Autodesk Inventor part; units mm, degrees
(part 2 of 2)
  spline S266 degree 2 poles (-40.3504, -60.3265) (-40.034, -60.3265) (-39.4952, -60.2771) (-39.3469, -60.198) knots 0 0 0 1 2 2 2
  spline S267 degree 2 poles (-39.3469, -60.198) (-39.1838, -60.1189) (-39.0256, -59.8173) (-39.0256, -59.5553) knots 0 0 0 1 2 2 2
  spline S268 degree 2 poles (-39.0256, -59.5553) (-39.0256, -59.3181) (-39.3173, -58.7743) (-39.5941, -58.4876) knots 0 0 0 1 2 2 2
  spline S269 degree 2 poles (-39.5941, -58.4876) (-39.6633, -58.4925) (-39.8561, -58.5024) (-39.9846, -58.5024) knots 0 0 0 1 2 2 2
  line L190 (-39.9846, -58.5024) -> (-43, -58.5024)
  line L191 (-43, -58.5024) -> (-43, -57.7313)
  line L192 (-43, -57.7313) -> (-40.3504, -57.7313)
  spline S270 degree 2 poles (-40.3504, -57.7313) (-40.034, -57.7313) (-39.4952, -57.6818) (-39.3469, -57.6028) knots 0 0 0 1 2 2 2
  spline S271 degree 2 poles (-39.3469, -57.6028) (-39.1838, -57.5237) (-39.0256, -57.2221) (-39.0256, -56.9601) knots 0 0 0 1 2 2 2
  spline S272 degree 2 poles (-39.0256, -56.9601) (-39.0256, -56.713) (-39.337, -56.1643) (-39.5793, -55.9072) knots 0 0 0 1 2 2 2
  line L193 (-39.5793, -55.9072) -> (-43, -55.9072)
  line L194 (-43, -55.9072) -> (-43, -55.1361)
  line L195 (-43, -55.1361) -> (-38.4225, -55.1361)
  line L196 (-38.4225, -55.1361) -> (-38.4225, -55.9072)
  line L197 (-38.4225, -55.9072) -> (-38.9267, -55.9072)
  spline S273 degree 2 poles (-38.9267, -55.9072) (-38.6252, -56.2088) (-38.294, -56.8019) (-38.294, -57.1579) knots 0 0 0 1 2 2 2
  spline S274 degree 2 poles (-38.294, -57.1579) (-38.294, -57.5632) (-38.6647, -58.191) (-39.0849, -58.3541) knots 0 0 0 1 2 2 2
  spline S275 degree 2 poles (-39.0849, -58.3541) (-38.6944, -58.7051) (-38.294, -59.3675) (-38.294, -59.7531) knots 0 0 0 1 2 2 2
  spline S276 degree 2 poles (-38.294, -59.7531) (-38.294, -60.0497) (-38.4769, -60.5341) (-38.6845, -60.7121) knots 0 0 0 1 2 2 2
  spline S277 degree 2 poles (-38.6845, -60.7121) (-38.8921, -60.895) (-39.515, -61.0976) (-39.9846, -61.0976) knots 0 0 0 1 2 2 2
  line L198 (-39.9846, -61.0976) -> (-43, -61.0976)
  line L199 (-43, -61.0976) -> (-43, -60.3265)
  spline S278 degree 2 poles (-53.1384, -40.6671) (-53.1384, -40.2123) (-52.8665, -39.4659) (-52.6144, -39.2039) knots 0 0 0 1 2 2 2
  spline S279 degree 2 poles (-52.6144, -39.2039) (-52.3673, -38.9468) (-51.695, -38.6799) (-51.3143, -38.6799) knots 0 0 0 1 2 2 2
  spline S280 degree 2 poles (-51.3143, -38.6799) (-50.82, -38.6799) (-49.9895, -39.2088) (-49.7424, -39.713) knots 0 0 0 1 2 2 2
  line L200 (-49.7424, -39.713) -> (-49.7177, -39.713)
  spline S281 degree 2 poles (-49.7177, -39.713) (-49.4557, -39.2632) (-48.8328, -38.8282) (-48.3682, -38.8282) knots 0 0 0 1 2 2 2
  spline S282 degree 2 poles (-48.3682, -38.8282) (-47.681, -38.8282) (-46.7616, -39.8663) (-46.7616, -40.6671) knots 0 0 0 1 2 2 2
  spline S283 degree 2 poles (-46.7616, -40.6671) (-46.7616, -41.4976) (-47.6316, -42.5011) (-48.3138, -42.5011) knots 0 0 0 1 2 2 2
  spline S284 degree 2 poles (-48.3138, -42.5011) (-48.7241, -42.5011) (-49.5249, -42.0216) (-49.7523, -41.5717) knots 0 0 0 1 2 2 2
  line L201 (-49.7523, -41.5717) -> (-49.777, -41.5717)
  spline S285 degree 2 poles (-49.777, -41.5717) (-50.0241, -42.1056) (-50.736, -42.6543) (-51.2995, -42.6543) knots 0 0 0 1 2 2 2
  spline S286 degree 2 poles (-51.2995, -42.6543) (-52.0806, -42.6543) (-53.1384, -41.5173) (-53.1384, -40.6671) knots 0 0 0 1 2 2 2
  spline S287 degree 2 poles (-51.3786, -41.8139) (-51.0029, -41.8139) (-50.558, -41.5173) (-50.3306, -41.0972) knots 0 0 0 1 2 2 2
  spline S288 degree 2 poles (-50.3306, -41.0972) (-50.2515, -40.9588) (-50.0686, -40.4941) (-49.95, -40.2024) knots 0 0 0 1 2 2 2
  spline S289 degree 2 poles (-49.95, -40.2024) (-50.1724, -39.8663) (-50.8348, -39.5054) (-51.255, -39.5054) knots 0 0 0 1 2 2 2
  spline S290 degree 2 poles (-51.255, -39.5054) (-51.8087, -39.5054) (-52.5304, -40.1728) (-52.5304, -40.677) knots 0 0 0 1 2 2 2
  spline S291 degree 2 poles (-52.5304, -40.677) (-52.5304, -41.1911) (-51.9125, -41.8139) (-51.3786, -41.8139) knots 0 0 0 1 2 2 2
  spline S292 degree 2 poles (-48.3237, -41.7002) (-47.9134, -41.7002) (-47.3647, -41.1515) (-47.3647, -40.6622) knots 0 0 0 1 2 2 2
  spline S293 degree 2 poles (-47.3647, -40.6622) (-47.3647, -40.2173) (-47.8541, -39.6488) (-48.2742, -39.6488) knots 0 0 0 1 2 2 2
  spline S294 degree 2 poles (-48.2742, -39.6488) (-48.5758, -39.6488) (-48.9959, -39.9404) (-49.164, -40.2321) knots 0 0 0 1 2 2 2
  spline S295 degree 2 poles (-49.164, -40.2321) (-49.2332, -40.3557) (-49.4754, -40.8797) (-49.5447, -41.0922) knots 0 0 0 1 2 2 2
  spline S296 degree 2 poles (-49.5447, -41.0922) (-49.2728, -41.4481) (-48.6944, -41.7002) (-48.3237, -41.7002) knots 0 0 0 1 2 2 2
  spline S297 degree 2 poles (-49.95, -47.1972) (-51.5912, -47.1972) (-53.1285, -46.2431) (-53.1285, -45.2495) knots 0 0 0 1 2 2 2
  spline S298 degree 2 poles (-53.1285, -45.2495) (-53.1285, -44.2411) (-51.5615, -43.2969) (-49.9549, -43.2969) knots 0 0 0 1 2 2 2
  spline S299 degree 2 poles (-49.9549, -43.2969) (-48.3039, -43.2969) (-46.7764, -44.251) (-46.7764, -45.2495) knots 0 0 0 1 2 2 2
  spline S300 degree 2 poles (-46.7764, -45.2495) (-46.7764, -46.253) (-48.3583, -47.1972) (-49.95, -47.1972) knots 0 0 0 1 2 2 2
  spline S301 degree 2 poles (-51.8087, -46.1492) (-51.5071, -46.2678) (-50.5778, -46.3667) (-49.95, -46.3667) knots 0 0 0 1 2 2 2
  spline S302 degree 2 poles (-49.95, -46.3667) (-49.3222, -46.3667) (-48.3978, -46.2678) (-48.0864, -46.1442) knots 0 0 0 1 2 2 2
  spline S303 degree 2 poles (-48.0864, -46.1442) (-47.775, -46.0207) (-47.4536, -45.5906) (-47.4536, -45.2495) knots 0 0 0 1 2 2 2
  spline S304 degree 2 poles (-47.4536, -45.2495) (-47.4536, -44.9084) (-47.775, -44.4685) (-48.0963, -44.34) knots 0 0 0 1 2 2 2
  spline S305 degree 2 poles (-48.0963, -44.34) (-48.4077, -44.2164) (-49.3568, -44.1274) (-49.9549, -44.1274) knots 0 0 0 1 2 2 2
  spline S306 degree 2 poles (-49.9549, -44.1274) (-50.5976, -44.1274) (-51.4577, -44.2065) (-51.7938, -44.335) knots 0 0 0 1 2 2 2
  spline S307 degree 2 poles (-51.7938, -44.335) (-52.1102, -44.4536) (-52.4513, -44.8936) (-52.4513, -45.2495) knots 0 0 0 1 2 2 2
  spline S308 degree 2 poles (-52.4513, -45.2495) (-52.4513, -45.5857) (-52.13, -46.0256) (-51.8087, -46.1492) knots 0 0 0 1 2 2 2
  line L202 (-53, -53.2823) -> (-50.3504, -53.2823)
  spline S309 degree 2 poles (-50.3504, -53.2823) (-50.034, -53.2823) (-49.4952, -53.2329) (-49.3469, -53.1538) knots 0 0 0 1 2 2 2
  spline S310 degree 2 poles (-49.3469, -53.1538) (-49.1838, -53.0747) (-49.0256, -52.7732) (-49.0256, -52.5112) knots 0 0 0 1 2 2 2
  spline S311 degree 2 poles (-49.0256, -52.5112) (-49.0256, -52.2739) (-49.3173, -51.7301) (-49.5941, -51.4434) knots 0 0 0 1 2 2 2
  spline S312 degree 2 poles (-49.5941, -51.4434) (-49.6633, -51.4484) (-49.8561, -51.4583) (-49.9846, -51.4583) knots 0 0 0 1 2 2 2
  line L203 (-49.9846, -51.4583) -> (-53, -51.4583)
  line L204 (-53, -51.4583) -> (-53, -50.6871)
  line L205 (-53, -50.6871) -> (-50.3504, -50.6871)
  spline S313 degree 2 poles (-50.3504, -50.6871) (-50.034, -50.6871) (-49.4952, -50.6377) (-49.3469, -50.5586) knots 0 0 0 1 2 2 2
  spline S314 degree 2 poles (-49.3469, -50.5586) (-49.1838, -50.4795) (-49.0256, -50.178) (-49.0256, -49.916) knots 0 0 0 1 2 2 2
  spline S315 degree 2 poles (-49.0256, -49.916) (-49.0256, -49.6688) (-49.337, -49.1201) (-49.5793, -48.863) knots 0 0 0 1 2 2 2
  line L206 (-49.5793, -48.863) -> (-53, -48.863)
  line L207 (-53, -48.863) -> (-53, -48.0919)
  line L208 (-53, -48.0919) -> (-48.4225, -48.0919)
  line L209 (-48.4225, -48.0919) -> (-48.4225, -48.863)
  line L210 (-48.4225, -48.863) -> (-48.9267, -48.863)
  spline S316 degree 2 poles (-48.9267, -48.863) (-48.6252, -49.1646) (-48.294, -49.7578) (-48.294, -50.1137) knots 0 0 0 1 2 2 2
  spline S317 degree 2 poles (-48.294, -50.1137) (-48.294, -50.519) (-48.6647, -51.1468) (-49.0849, -51.31) knots 0 0 0 1 2 2 2
  spline S318 degree 2 poles (-49.0849, -51.31) (-48.6944, -51.6609) (-48.294, -52.3233) (-48.294, -52.7089) knots 0 0 0 1 2 2 2
  spline S319 degree 2 poles (-48.294, -52.7089) (-48.294, -53.0055) (-48.4769, -53.49) (-48.6845, -53.6679) knots 0 0 0 1 2 2 2
  spline S320 degree 2 poles (-48.6845, -53.6679) (-48.8921, -53.8508) (-49.515, -54.0535) (-49.9846, -54.0535) knots 0 0 0 1 2 2 2
  line L211 (-49.9846, -54.0535) -> (-53, -54.0535)
  line L212 (-53, -54.0535) -> (-53, -53.2823)
  line L213 (-53, -60.3265) -> (-50.3504, -60.3265)
  spline S321 degree 2 poles (-50.3504, -60.3265) (-50.034, -60.3265) (-49.4952, -60.2771) (-49.3469, -60.198) knots 0 0 0 1 2 2 2
  spline S322 degree 2 poles (-49.3469, -60.198) (-49.1838, -60.1189) (-49.0256, -59.8173) (-49.0256, -59.5553) knots 0 0 0 1 2 2 2
  spline S323 degree 2 poles (-49.0256, -59.5553) (-49.0256, -59.3181) (-49.3173, -58.7743) (-49.5941, -58.4876) knots 0 0 0 1 2 2 2
  spline S324 degree 2 poles (-49.5941, -58.4876) (-49.6633, -58.4925) (-49.8561, -58.5024) (-49.9846, -58.5024) knots 0 0 0 1 2 2 2
  line L214 (-49.9846, -58.5024) -> (-53, -58.5024)
  line L215 (-53, -58.5024) -> (-53, -57.7313)
  line L216 (-53, -57.7313) -> (-50.3504, -57.7313)
  spline S325 degree 2 poles (-50.3504, -57.7313) (-50.034, -57.7313) (-49.4952, -57.6818) (-49.3469, -57.6028) knots 0 0 0 1 2 2 2
  spline S326 degree 2 poles (-49.3469, -57.6028) (-49.1838, -57.5237) (-49.0256, -57.2221) (-49.0256, -56.9601) knots 0 0 0 1 2 2 2
  spline S327 degree 2 poles (-49.0256, -56.9601) (-49.0256, -56.713) (-49.337, -56.1643) (-49.5793, -55.9072) knots 0 0 0 1 2 2 2
  line L217 (-49.5793, -55.9072) -> (-53, -55.9072)
  line L218 (-53, -55.9072) -> (-53, -55.1361)
  line L219 (-53, -55.1361) -> (-48.4225, -55.1361)
  line L220 (-48.4225, -55.1361) -> (-48.4225, -55.9072)
  line L221 (-48.4225, -55.9072) -> (-48.9267, -55.9072)
  spline S328 degree 2 poles (-48.9267, -55.9072) (-48.6252, -56.2088) (-48.294, -56.8019) (-48.294, -57.1579) knots 0 0 0 1 2 2 2
  spline S329 degree 2 poles (-48.294, -57.1579) (-48.294, -57.5632) (-48.6647, -58.191) (-49.0849, -58.3541) knots 0 0 0 1 2 2 2
  spline S330 degree 2 poles (-49.0849, -58.3541) (-48.6944, -58.7051) (-48.294, -59.3675) (-48.294, -59.7531) knots 0 0 0 1 2 2 2
  spline S331 degree 2 poles (-48.294, -59.7531) (-48.294, -60.0497) (-48.4769, -60.5341) (-48.6845, -60.7121) knots 0 0 0 1 2 2 2
  spline S332 degree 2 poles (-48.6845, -60.7121) (-48.8921, -60.895) (-49.515, -61.0976) (-49.9846, -61.0976) knots 0 0 0 1 2 2 2
  line L222 (-49.9846, -61.0976) -> (-53, -61.0976)
  line L223 (-53, -61.0976) -> (-53, -60.3265)
  spline S333 degree 2 poles (-58.8823, -38.6552) (-58.4126, -38.6552) (-57.6316, -38.9617) (-57.3498, -39.2286) knots 0 0 0 1 2 2 2
  spline S334 degree 2 poles (-57.3498, -39.2286) (-57.078, -39.4807) (-56.7764, -40.2173) (-56.7764, -40.5929) knots 0 0 0 1 2 2 2
  spline S335 degree 2 poles (-56.7764, -40.5929) (-56.7764, -41.0131) (-57.0582, -41.6953) (-57.3251, -41.9474) knots 0 0 0 1 2 2 2
  spline S336 degree 2 poles (-57.3251, -41.9474) (-57.6613, -42.2638) (-58.7488, -42.6098) (-59.5842, -42.6098) knots 0 0 0 1 2 2 2
  spline S337 degree 2 poles (-59.5842, -42.6098) (-60.3405, -42.6098) (-61.695, -42.2687) (-62.1448, -41.9375) knots 0 0 0 1 2 2 2
  spline S338 degree 2 poles (-62.1448, -41.9375) (-62.6194, -41.5865) (-63.1186, -40.5979) (-63.1186, -39.8762) knots 0 0 0 1 2 2 2
  spline S339 degree 2 poles (-63.1186, -39.8762) (-63.1186, -39.713) (-63.084, -39.3423) (-63.0346, -39.1841) knots 0 0 0 1 2 2 2
  line L224 (-63.0346, -39.1841) -> (-62.2486, -39.1841)
  line L225 (-62.2486, -39.1841) -> (-62.2486, -39.2237)
  spline S340 degree 2 poles (-62.2486, -39.2237) (-62.3079, -39.3275) (-62.4118, -39.7625) (-62.4118, -39.9849) knots 0 0 0 1 2 2 2
  spline S341 degree 2 poles (-62.4118, -39.9849) (-62.4118, -40.7857) (-61.3539, -41.7002) (-60.3751, -41.7645) knots 0 0 0 1 2 2 2
  spline S342 degree 2 poles (-60.3751, -41.7645) (-60.5976, -41.4382) (-60.8002, -40.8451) (-60.8002, -40.4941) knots 0 0 0 1 2 2 2
  spline S343 degree 2 poles (-60.8002, -40.4941) (-60.8002, -40.1579) (-60.6519, -39.5994) (-60.4394, -39.3176) knots 0 0 0 1 2 2 2
  spline S344 degree 2 poles (-60.4394, -39.3176) (-60.1873, -38.9913) (-59.4211, -38.6552) (-58.8823, -38.6552) knots 0 0 0 1 2 2 2
  spline S345 degree 2 poles (-59.4013, -41.7843) (-58.7834, -41.7843) (-58.0023, -41.5569) (-57.7898, -41.3542) knots 0 0 0 1 2 2 2
  spline S346 degree 2 poles (-57.7898, -41.3542) (-57.5921, -41.1763) (-57.4438, -40.8055) (-57.4438, -40.588) knots 0 0 0 1 2 2 2
  spline S347 degree 2 poles (-57.4438, -40.588) (-57.4438, -40.0838) (-58.1655, -39.4857) (-58.8476, -39.4857) knots 0 0 0 1 2 2 2
  spline S348 degree 2 poles (-58.8476, -39.4857) (-59.2332, -39.4857) (-59.7325, -39.6834) (-59.9105, -39.9009) knots 0 0 0 1 2 2 2
  spline S349 degree 2 poles (-59.9105, -39.9009) (-60.039, -40.0591) (-60.123, -40.4496) (-60.123, -40.677) knots 0 0 0 1 2 2 2
  spline S350 degree 2 poles (-60.123, -40.677) (-60.123, -40.939) (-59.9401, -41.5421) (-59.7869, -41.7694) knots 0 0 0 1 2 2 2
  spline S351 degree 2 poles (-59.7869, -41.7694) (-59.7276, -41.7744) (-59.5249, -41.7843) (-59.4013, -41.7843) knots 0 0 0 1 2 2 2
  spline S352 degree 2 poles (-59.95, -47.1972) (-61.5912, -47.1972) (-63.1285, -46.2431) (-63.1285, -45.2495) knots 0 0 0 1 2 2 2
  spline S353 degree 2 poles (-63.1285, -45.2495) (-63.1285, -44.2411) (-61.5615, -43.2969) (-59.9549, -43.2969) knots 0 0 0 1 2 2 2
  spline S354 degree 2 poles (-59.9549, -43.2969) (-58.3039, -43.2969) (-56.7764, -44.251) (-56.7764, -45.2495) knots 0 0 0 1 2 2 2
  spline S355 degree 2 poles (-56.7764, -45.2495) (-56.7764, -46.253) (-58.3583, -47.1972) (-59.95, -47.1972) knots 0 0 0 1 2 2 2
  spline S356 degree 2 poles (-61.8087, -46.1492) (-61.5071, -46.2678) (-60.5778, -46.3667) (-59.95, -46.3667) knots 0 0 0 1 2 2 2
  spline S357 degree 2 poles (-59.95, -46.3667) (-59.3222, -46.3667) (-58.3978, -46.2678) (-58.0864, -46.1442) knots 0 0 0 1 2 2 2
  spline S358 degree 2 poles (-58.0864, -46.1442) (-57.775, -46.0207) (-57.4536, -45.5906) (-57.4536, -45.2495) knots 0 0 0 1 2 2 2
  spline S359 degree 2 poles (-57.4536, -45.2495) (-57.4536, -44.9084) (-57.775, -44.4685) (-58.0963, -44.34) knots 0 0 0 1 2 2 2
  spline S360 degree 2 poles (-58.0963, -44.34) (-58.4077, -44.2164) (-59.3568, -44.1274) (-59.9549, -44.1274) knots 0 0 0 1 2 2 2
  spline S361 degree 2 poles (-59.9549, -44.1274) (-60.5976, -44.1274) (-61.4577, -44.2065) (-61.7938, -44.335) knots 0 0 0 1 2 2 2
  spline S362 degree 2 poles (-61.7938, -44.335) (-62.1102, -44.4536) (-62.4513, -44.8936) (-62.4513, -45.2495) knots 0 0 0 1 2 2 2
  spline S363 degree 2 poles (-62.4513, -45.2495) (-62.4513, -45.5857) (-62.13, -46.0256) (-61.8087, -46.1492) knots 0 0 0 1 2 2 2
  line L226 (-63, -53.2823) -> (-60.3504, -53.2823)
  spline S364 degree 2 poles (-60.3504, -53.2823) (-60.034, -53.2823) (-59.4952, -53.2329) (-59.3469, -53.1538) knots 0 0 0 1 2 2 2
  spline S365 degree 2 poles (-59.3469, -53.1538) (-59.1838, -53.0747) (-59.0256, -52.7732) (-59.0256, -52.5112) knots 0 0 0 1 2 2 2
  spline S366 degree 2 poles (-59.0256, -52.5112) (-59.0256, -52.2739) (-59.3173, -51.7301) (-59.5941, -51.4434) knots 0 0 0 1 2 2 2
  spline S367 degree 2 poles (-59.5941, -51.4434) (-59.6633, -51.4484) (-59.8561, -51.4583) (-59.9846, -51.4583) knots 0 0 0 1 2 2 2
  line L227 (-59.9846, -51.4583) -> (-63, -51.4583)
  line L228 (-63, -51.4583) -> (-63, -50.6871)
  line L229 (-63, -50.6871) -> (-60.3504, -50.6871)
  spline S368 degree 2 poles (-60.3504, -50.6871) (-60.034, -50.6871) (-59.4952, -50.6377) (-59.3469, -50.5586) knots 0 0 0 1 2 2 2
  spline S369 degree 2 poles (-59.3469, -50.5586) (-59.1838, -50.4795) (-59.0256, -50.178) (-59.0256, -49.916) knots 0 0 0 1 2 2 2
  spline S370 degree 2 poles (-59.0256, -49.916) (-59.0256, -49.6688) (-59.337, -49.1201) (-59.5793, -48.863) knots 0 0 0 1 2 2 2
  line L230 (-59.5793, -48.863) -> (-63, -48.863)
  line L231 (-63, -48.863) -> (-63, -48.0919)
  line L232 (-63, -48.0919) -> (-58.4225, -48.0919)
  line L233 (-58.4225, -48.0919) -> (-58.4225, -48.863)
  line L234 (-58.4225, -48.863) -> (-58.9267, -48.863)
  spline S371 degree 2 poles (-58.9267, -48.863) (-58.6252, -49.1646) (-58.294, -49.7578) (-58.294, -50.1137) knots 0 0 0 1 2 2 2
  spline S372 degree 2 poles (-58.294, -50.1137) (-58.294, -50.519) (-58.6647, -51.1468) (-59.0849, -51.31) knots 0 0 0 1 2 2 2
  spline S373 degree 2 poles (-59.0849, -51.31) (-58.6944, -51.6609) (-58.294, -52.3233) (-58.294, -52.7089) knots 0 0 0 1 2 2 2
  spline S374 degree 2 poles (-58.294, -52.7089) (-58.294, -53.0055) (-58.4769, -53.49) (-58.6845, -53.6679) knots 0 0 0 1 2 2 2
  spline S375 degree 2 poles (-58.6845, -53.6679) (-58.8921, -53.8508) (-59.515, -54.0535) (-59.9846, -54.0535) knots 0 0 0 1 2 2 2
  line L235 (-59.9846, -54.0535) -> (-63, -54.0535)
  line L236 (-63, -54.0535) -> (-63, -53.2823)
  line L237 (-63, -60.3265) -> (-60.3504, -60.3265)
  spline S376 degree 2 poles (-60.3504, -60.3265) (-60.034, -60.3265) (-59.4952, -60.2771) (-59.3469, -60.198) knots 0 0 0 1 2 2 2
  spline S377 degree 2 poles (-59.3469, -60.198) (-59.1838, -60.1189) (-59.0256, -59.8173) (-59.0256, -59.5553) knots 0 0 0 1 2 2 2
  spline S378 degree 2 poles (-59.0256, -59.5553) (-59.0256, -59.3181) (-59.3173, -58.7743) (-59.5941, -58.4876) knots 0 0 0 1 2 2 2
  spline S379 degree 2 poles (-59.5941, -58.4876) (-59.6633, -58.4925) (-59.8561, -58.5024) (-59.9846, -58.5024) knots 0 0 0 1 2 2 2
  line L238 (-59.9846, -58.5024) -> (-63, -58.5024)
  line L239 (-63, -58.5024) -> (-63, -57.7313)
  line L240 (-63, -57.7313) -> (-60.3504, -57.7313)
  spline S380 degree 2 poles (-60.3504, -57.7313) (-60.034, -57.7313) (-59.4952, -57.6818) (-59.3469, -57.6028) knots 0 0 0 1 2 2 2
  spline S381 degree 2 poles (-59.3469, -57.6028) (-59.1838, -57.5237) (-59.0256, -57.2221) (-59.0256, -56.9601) knots 0 0 0 1 2 2 2
  spline S382 degree 2 poles (-59.0256, -56.9601) (-59.0256, -56.713) (-59.337, -56.1643) (-59.5793, -55.9072) knots 0 0 0 1 2 2 2
  line L241 (-59.5793, -55.9072) -> (-63, -55.9072)
  line L242 (-63, -55.9072) -> (-63, -55.1361)
  line L243 (-63, -55.1361) -> (-58.4225, -55.1361)
  line L244 (-58.4225, -55.1361) -> (-58.4225, -55.9072)
  line L245 (-58.4225, -55.9072) -> (-58.9267, -55.9072)
  spline S383 degree 2 poles (-58.9267, -55.9072) (-58.6252, -56.2088) (-58.294, -56.8019) (-58.294, -57.1579) knots 0 0 0 1 2 2 2
  spline S384 degree 2 poles (-58.294, -57.1579) (-58.294, -57.5632) (-58.6647, -58.191) (-59.0849, -58.3541) knots 0 0 0 1 2 2 2
  spline S385 degree 2 poles (-59.0849, -58.3541) (-58.6944, -58.7051) (-58.294, -59.3675) (-58.294, -59.7531) knots 0 0 0 1 2 2 2
  spline S386 degree 2 poles (-58.294, -59.7531) (-58.294, -60.0497) (-58.4769, -60.5341) (-58.6845, -60.7121) knots 0 0 0 1 2 2 2
  spline S387 degree 2 poles (-58.6845, -60.7121) (-58.8921, -60.895) (-59.515, -61.0976) (-59.9846, -61.0976) knots 0 0 0 1 2 2 2
  line L246 (-59.9846, -61.0976) -> (-63, -61.0976)
  line L247 (-63, -61.0976) -> (-63, -60.3265)
  point P0 (0, 0)
  dimension "d20" = 20
  constraints: 16 end point, 13 vertical, 3 parallel
  measures "d20" distance from line of A3.centre L2
emboss "Emboss1" sketch "Sketch4" operation cut depth 1 direction (0, 0, -1)
equation "\"d11\" = d10"
equation "\"d12\" = d10"
equation "\"d13\" = d10"
equation "\"d14\" = d10"
body "Solid1"
